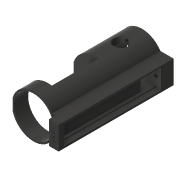
# Autodesk Inventor part: Holder for Fan
Saved by Autodesk Inventor 2017 (Build 210142000, 142)
## iProperties
Created: 2016-08-05
Part Number: Holder for Fan
Material: Generic
Document SubType Name: Modeling
Designer: ge937963
Density: 1 g/cm^3
Appearance: Smooth - Black
Mass: 19.5936 g
Surface Area: 136.055 cm^2
Volume: 19.5936 cm^3
Author: ge937963
Autodesk Inventor part; units mm, degrees
ref_plane "YZ Plane" through (0, 0, 0) normal (1, 0, 0) x (0, 1, 0)
ref_plane "XZ Plane" through (0, 0, 0) normal (0, 1, 0) x (-1, 0, 0)
sketch "Sketch1" plane through (0, 0, 0) normal (0, 0, 1) x (1, 0, 0)
  circle A0 centre (0, 0) radius 12.7
  circle A1 centre (0, 0) radius 9.525
  dimension "d0" = 25.4
  dimension "d1" = 19.05
  constraints: 2 centre point, 2 coincident
  measures "d0" diameter of A0
  measures "d1" diameter of A1
extrude "Extrusion1" add sketch "Sketch1" along normal blind 25.4 and the other way blind 12.7
sketch "Sketch2" plane through (0, 0, -12.7) normal (0, 0, -1) x (-1, 0, 0)
  circle A0 centre (0, 0) radius 12.7
  dimension "d6" = 25.4
  constraints: 1 centre point, 1 coincident
  measures "d6" diameter of A0
extrude "Extrusion2" add sketch "Sketch2" against normal blind 3.175
sketch "Sketch3" plane through (0, 0, -12.7) normal (0, 0, -1) x (-1, 0, 0)
  circle A0 centre (0, 0) radius 14.2875
  circle A1 centre (0, 0) radius 12.7
  dimension "d9" = 28.575
  constraints: 2 centre point, 2 coincident
  measures "d9" diameter of A0
extrude "Extrusion3" add sketch "Sketch3" against normal blind 66.675
sketch "Sketch4" plane through (0, 0, 0) normal (1, 0, 0) x (0, 1, 0)
  line L0 (-19.206, 6.35) -> (20.1125, 6.35)
  line L1 (20.1125, 6.35) -> (20.1125, 25.4)
  line L2 (20.1125, 25.4) -> (-19.206, 25.4)
  line L3 (-19.206, 25.4) -> (-19.206, 6.35)
  line L4 (14.2875, -12.7) -> (-14.2875, -12.7) projected
  point P0 (0, 0)
  dimension "d12" = 19.05
  dimension "d13" = 19.05
  constraints: 8 end point, 2 parallel, 1 horizontal, 1 perpendicular
  measures "d12" distance of L0.end L1.end
  measures "d13" distance from line of L4 L0.end
extrude "Extrusion4" cut sketch "Sketch4" along normal blind 2.54 and the other way blind 66.675
sketch "Sketch5" plane through (0, 0, 0) normal (1, 0, 0) x (0, 1, 0)
  line L0 (-1.5875, -17.2077) -> (1.5875, -17.2077) projected
  line L1 (-1.5875, -18.0015) -> (-1.5875, -16.414) projected
  line L2 (1.5875, -16.414) -> (-1.5875, -16.414) projected
  line L3 (1.5875, -16.414) -> (1.5875, -18.0015) projected
  line L4 (-1.5875, -18.0015) -> (1.5875, -18.0015) projected
  line L5 (-1.7071, -16.2944) -> (-1.7071, -18.121)
  line L6 (-1.7071, -18.121) -> (1.7071, -18.121)
  line L7 (1.7071, -18.121) -> (1.7071, -16.2944)
  line L8 (1.7071, -16.2944) -> (-1.7071, -16.2944)
  point P0 (0, 0)
  constraints: 8 end point, 3 other
extrude "Extrusion5" cut sketch "Sketch5" along normal blind 66.675 contours L1 L2 L3 L0 | L0 L3 L4 L1 | L8 L7 L6 L5
sketch "Sketch6" plane through (0, 0, 53.975) normal (0, 0, 1) x (1, 0, 0)
  line L0 (19.2175, 5.4663) -> (15.9155, 5.4663) projected
  line L1 (15.9155, 5.4663) -> (15.9155, -5.4557) projected
  line L2 (15.9155, -5.4557) -> (19.2175, -5.4557) projected
  line L3 (19.2175, -5.4557) -> (19.2175, 5.4663) projected
  line L4 (20.7415, -7.6147) -> (14.3915, -7.6147) projected
  line L5 (14.3915, -7.6147) -> (14.3915, 7.6253) projected
  line L6 (14.3915, 7.6253) -> (20.7415, 7.6253) projected
  line L7 (20.7415, 7.6253) -> (20.7415, -7.6147) projected
  point P0 (0, 0)
extrude "Extrusion6" add sketch "Sketch6" against normal blind 9.525
sketch "Sketch7" plane through (14.3915, -7.6147, 53.975) normal (-1, 0, 0) x (0, 0, 1)
  line L0 (0, 0) -> (0, 15.24) projected
  line L1 (0, 15.24) -> (-9.525, 15.24) projected
  line L2 (-9.525, 0) -> (-9.525, 15.24) projected
  line L3 (0, 0) -> (-9.525, 0) projected
  point P0 (-53.975, 7.6147)
extrude "Extrusion7" add sketch "Sketch7" along normal blind 2.54
sketch "Sketch8" plane through (0, 0, 53.975) normal (0, 0, 1) x (1, 0, 0)
  arc A0 (11.8515, 4.5641) -> (11.8515, -4.5641) centre (0, 0) ccw projected
  arc A1 (2.54, -12.4434) -> (2.54, 12.4434) centre (0, 0) ccw projected
  point P0 (0, -12.7)
  point P1 (0, 12.7)
extrude "Extrusion8" cut sketch "Sketch8" against normal blind 12.7
sketch "Sketch9" plane through (0, 0, 44.45) normal (0, 0, -1) x (-1, 0, 0)
  line L0 (-15.9155, 5.4663) -> (-15.9155, -5.4557) projected
  line L1 (-15.9155, -5.4557) -> (-19.2175, -5.4557) projected
  line L2 (-19.2175, -5.4557) -> (-19.2175, 5.4663) projected
  line L3 (-19.2175, 5.4663) -> (-15.9155, 5.4663) projected
  line L4 (-20.7415, -7.6147) -> (-12.0892, -7.6147) projected
  arc A0 (-12.0826, 7.6253) -> (-12.0892, -7.6147) centre (0, 0) ccw projected
  line L5 (-20.7415, 7.6253) -> (-12.0826, 7.6253) projected
  line L6 (-20.7415, 7.6253) -> (-20.7415, -7.6147) projected
extrude "Extrusion9" add sketch "Sketch9" along normal up to surface (57.15 mm away)
sketch "Sketch10" plane through (0, 0, -12.7) normal (0, 0, -1) x (-1, 0, 0)
  line L0 (-15.9155, 5.4663) -> (-15.9155, -5.4557) projected
  line L1 (-19.2175, -5.4557) -> (-19.2175, 5.4663) projected
  line L2 (-15.9155, 5.4663) -> (-19.2175, 5.4663)
  line L3 (-19.2175, 5.4663) -> (-19.2175, -5.4557)
  line L4 (-19.2175, -5.4557) -> (-15.9155, -5.4557)
  line L5 (-15.9155, -5.4557) -> (-15.9155, 5.4663)
  point P0 (0, 0)
  constraints: 8 end point, 2 parallel, 1 horizontal, 1 perpendicular
extrude "Extrusion10" add sketch "Sketch10" against normal blind 3.175
sketch "Sketch11" plane through (20.7415, -7.6147, 53.975) normal (1, 0, 0) x (0, 0, -1)
  line L0 (0, 15.24) -> (0, 0) projected
  line L1 (0, 0) -> (66.675, 0) projected
  line L2 (66.675, 15.24) -> (66.675, 0) projected
  line L3 (0, 15.24) -> (66.675, 15.24) projected
  line L4 (0, 1.27) -> (63.5, 1.27)
  line L5 (63.5, 1.27) -> (63.5, 13.97)
  line L6 (63.5, 13.97) -> (0, 13.97)
  line L7 (0, 13.97) -> (0, 1.27)
  point P0 (53.975, 7.6147)
  dimension "d28" = 0
  dimension "d29" = 1.27
  dimension "d30" = 1.27
  dimension "d31" = 63.5
  constraints: 8 end point, 2 parallel, 1 horizontal, 1 perpendicular
  measures "d28" distance between parallel lines of L0 L7
  measures "d29" distance between parallel lines of L1 L4
  measures "d30" distance between parallel lines of L3 L6
  measures "d31" distance of L5.end L6.end
extrude "Extrusion11" cut sketch "Sketch11" against normal blind 3.175 contours L6 L5 L4 L0
sketch "Sketch12" plane through (0, 0, 53.975) normal (0, 0, 1) x (1, 0, 0)
  line L0 (19.2175, 5.4663) -> (15.9155, 5.4663) projected
  line L1 (15.9155, 5.4663) -> (15.9155, -5.4557) projected
  line L2 (15.9155, -5.4557) -> (19.2175, -5.4557) projected
  line L3 (19.2175, -5.4557) -> (19.2175, 5.4663) projected
  line L4 (20.7415, -7.6147) -> (14.3915, -7.6147) projected
  line L5 (14.3915, -7.6147) -> (14.3915, 7.6253) projected
  line L6 (14.3915, 7.6253) -> (20.7415, 7.6253) projected
  line L7 (20.7415, 7.6253) -> (20.7415, -7.6147) projected
  line L8 (14.3915, -7.6147) -> (20.7415, -7.6147) projected
  line L9 (20.7415, -7.6147) -> (20.7415, 7.6253) projected
  line L10 (20.7415, 7.6253) -> (14.3915, 7.6253) projected
  line L11 (14.3915, 7.6253) -> (14.3915, -7.6147) projected
  circle A0 centre (17.5665, 3.8153) radius 0.762 projected
  circle A1 centre (17.5665, 1.2753) radius 0.762 projected
  circle A2 centre (17.5665, -1.2647) radius 0.762 projected
  circle A3 centre (17.5665, -3.8047) radius 0.762 projected
  line L12 (17.5665, -6.3447) -> (17.5665, -5.4557) projected
  line L13 (17.5665, -5.4557) -> (17.5665, -6.3447) projected
  line L14 (17.5665, 6.3553) -> (17.5665, 5.4663) projected
  line L15 (17.5665, 5.4663) -> (17.5665, 6.3553) projected
  line L16 (17.5665, -5.4557) -> (15.9155, -5.4557) projected
  line L17 (17.5665, -5.4557) -> (15.9155, -5.4557)
  line L18 (15.9155, -5.4557) -> (15.9155, 5.4663) projected
  line L19 (15.9155, -5.4557) -> (15.9155, 5.4663)
  line L20 (15.9155, 5.4663) -> (17.5665, 5.4663)
  line L21 (17.5665, 6.3553) -> (17.5665, 5.4663) projected
  line L22 (17.5665, 6.3553) -> (20.7415, 6.3553)
  line L23 (20.7415, -6.3447) -> (17.5665, -6.3447)
  line L24 (20.7415, 7.6253) -> (20.7415, -7.6147) projected
  line L25 (17.5665, -5.4557) -> (17.5665, -6.3447) projected
  line L26 (17.5665, -5.4557) -> (15.9155, -5.4557)
  line L27 (20.7415, -6.3447) -> (20.7415, -7.6147)
  point P0 (0, 0)
  constraints: 14 end point, 5 perpendicular, 1 collinear, 1 parallel
extrude "Extrusion12" add sketch "Sketch12" along normal up to surface (4.1732 mm away) contours L0 L1 L2 L12 L23 L7 L4 L5 L6 L22 L14
sketch "Sketch13" plane through (15.9155, -5.4557, -9.525) normal (1, 0, 0) x (0, 0, -1)
  line L0 (3.175, -2.159) -> (-67.6732, -2.159) projected
  line L1 (-66.6572, -2.159) -> (-67.6732, -2.159)
  line L2 (-67.6732, -2.159) -> (-67.6732, 13.081)
  line L3 (-67.6732, 13.081) -> (-66.6572, 13.081)
  line L4 (-66.6572, 13.081) -> (-66.6572, -2.159)
  line L5 (-66.6572, 9.7155) -> (-72.4992, 9.7155)
  point P0 (-9.525, 5.4557)
  point P1 (-67.1652, -2.159)
  point P2 (-67.1652, 13.081)
  point P3 (-67.6732, 5.461)
  constraints: 10 end point, 3 midpoint, 2 horizontal, 2 horizontal alignment, 2 parallel, 2 vertical alignment, 1 perpendicular, 1 point on line, 2 other
extrude "Extrusion13" add sketch "Sketch13" along normal up to surface (4.826 mm away)
sketch "Sketch14" plane through (14.3915, 7.6253, 58.1482) normal (0, 0, 1) x (1, 0, 0)
  circle A0 centre (3.175, -3.81) radius 0.762 projected
  circle A1 centre (3.175, -6.35) radius 0.762 projected
  circle A2 centre (3.175, -8.89) radius 0.762 projected
  circle A3 centre (3.175, -11.43) radius 0.762 projected
  point P0 (-14.3915, -7.6253)
extrude "Extrusion14" cut sketch "Sketch14" against normal blind 3.175
sketch "Sketch15" plane through (17.5665, -7.6147, 53.975) normal (1, 0, 0) x (0, 0, -1)
  line L0 (2.1768, 15.24) -> (5.7328, 15.24) projected
  line L1 (2.1768, 0) -> (2.1768, 15.24) projected
  line L2 (5.7328, 0) -> (2.1768, 0) projected
  line L3 (5.7328, 15.24) -> (5.7328, 0) projected
  line L4 (-3.1572, 13.081) -> (5.7328, 13.081) projected
  line L5 (-3.1572, 2.159) -> (5.7328, 2.159) projected
  line L6 (63.5, 1.27) -> (-3.1572, 1.27) projected
  line L7 (-3.1572, 2.159) -> (5.7328, 2.159)
  line L8 (5.7328, 2.159) -> (5.7328, 1.27)
  line L9 (5.7328, 1.27) -> (-3.1572, 1.27)
  line L10 (-3.1572, 1.27) -> (-3.1572, 2.159)
  line L11 (-3.1572, 13.081) -> (-3.1572, 2.159) projected
  line L12 (-3.1572, 13.97) -> (63.5, 13.97) projected
  line L13 (-3.1572, 13.081) -> (5.7328, 13.081)
  line L14 (5.7328, 13.081) -> (5.7328, 13.97)
  line L15 (5.7328, 13.97) -> (-3.1572, 13.97)
  line L16 (-3.1572, 13.97) -> (-3.1572, 13.081)
  point P0 (53.975, 7.6147)
  constraints: 16 end point, 4 parallel, 4 point on line, 2 perpendicular, 1 horizontal
extrude "Extrusion15" add sketch "Sketch15" along normal up to surface (3.175 mm away) contours L12 L3 L4 L1 | L1 L4 L16 L12 | L5 L3 L6 L1 | L1 L6 L10 L5
sketch "Sketch16" plane through (15.9155, -5.4557, 57.1322) normal (0, 0, -1) x (-1, 0, 0)
  line L0 (-4.826, 10.922) -> (-4.826, 0) projected
  line L1 (-4.826, 10.922) -> (0, 10.922) projected
  line L2 (-4.826, 0) -> (-3.302, 0)
  line L3 (-3.302, 0) -> (-3.302, 10.922)
  line L4 (-3.302, 10.922) -> (-4.826, 10.922)
  line L5 (-4.826, 10.922) -> (-4.826, 0)
  line L6 (-3.302, 10.922) -> (-3.302, 0) projected
  point P0 (15.9155, 5.4557)
  point P1 (-3.302, 5.461)
  point P2 (-4.826, 11.811)
  point P3 (-4.826, -0.889)
  point P4 (-1.651, 10.922)
  constraints: 8 end point, 2 parallel, 1 collinear, 1 horizontal, 1 midpoint, 1 perpendicular, 1 point on line, 1 vertical alignment
ref_plane "Work Plane1" through (14.3915, -7.6147, 54.5922) normal (0, 0, -1) x (0, 1, 0)
extrude "Extrusion16" add sketch "Sketch16" along normal up to surface (2.54 mm away)
sketch "Sketch17" plane through (15.9155, -5.4557, -9.525) normal (1, 0, 0) x (0, 0, -1)
  line L0 (0, 2.2807) -> (-3.175, 2.2807)
  line L1 (-3.175, 2.2807) -> (-3.175, 8.6307)
  line L2 (-3.175, 8.6307) -> (0, 8.6307)
  line L3 (0, 8.6307) -> (0, 2.2807)
  line L4 (-66.6572, 10.922) -> (-66.6572, 0) projected
  line L5 (-66.6572, 0) -> (0, 0) projected
  line L6 (0, 0) -> (0, 10.922) projected
  line L7 (0, 10.922) -> (-66.6572, 10.922) projected
  point P0 (-9.525, 5.4557)
  point P1 (-3.175, 5.4557)
  dimension "d44" = 6.35
  dimension "d45" = 3.175
  dimension "d46" = 0
  constraints: 8 end point, 2 parallel, 1 horizontal, 1 horizontal alignment, 1 midpoint, 1 perpendicular
  measures "d44" distance of L0.end L1.end
  measures "d45" distance of L0.start L0.end
  measures "d46" distance between parallel lines of L6 L3
extrude "Extrusion17" cut sketch "Sketch17" against normal blind 12.7 contours L0 L1 L2 L3
sketch "Sketch18" plane through (0, 0, -12.7) normal (0, 0, -1) x (-1, 0, 0)
  line L0 (16.7262, -5.3355) -> (13.6621, -5.3355)
  line L1 (13.6621, -5.3355) -> (13.6621, 5.7627)
  line L2 (13.6621, 5.7627) -> (16.7262, 5.7627)
  line L3 (16.7262, 5.7627) -> (16.7262, -5.3355)
  point P0 (0, 0)
  constraints: 8 end point, 2 parallel, 1 horizontal, 1 perpendicular
extrude "Extrusion18" cut sketch "Sketch18" against normal through all
sketch "Sketch19" plane through (0, 0, 53.975) normal (0, 0, 1) x (1, 0, 0)
  circle A0 centre (0, 0) radius 13.208
  dimension "d51" = 26.416
  constraints: 1 centre point, 1 coincident
  measures "d51" diameter of A0
extrude "Extrusion19" cut sketch "Sketch19" against normal up to surface (28.575 mm away)
sketch "Sketch20" plane through (0, 0, 25.4) normal (0, 0, 1) x (1, 0, 0)
  circle A0 centre (0, 0) radius 10.033
  dimension "d54" = 20.066
  constraints: 1 centre point, 1 coincident
  measures "d54" diameter of A0
extrude "Extrusion20" cut sketch "Sketch20" against normal up to surface (34.925 mm away)
chamfer "Chamfer1" distance 3.175 angle 45 2 edges at (7.9418, 6.131, 25.4) (7.9418, -6.131, 25.4)
sketch "Sketch21" plane through (0, 0, -12.7) normal (0, 0, -1) x (-1, 0, 0)
  line L0 (13.6621, -4.1808) -> (13.6621, 4.1808) projected
  arc A0 (13.6621, 4.1808) -> (-12.0826, 7.6253) centre (0, 0) ccw projected
  line L1 (-12.0826, 7.6253) -> (-20.7415, 7.6253) projected
  line L2 (-20.7415, 7.6253) -> (-20.7415, -7.6147) projected
  line L3 (-20.7415, -7.6147) -> (-12.0892, -7.6147) projected
  arc A1 (-12.0892, -7.6147) -> (13.6621, -4.1808) centre (0, 0) ccw projected
extrude "Extrusion21" add sketch "Sketch21" along normal blind 5.08
chamfer "Chamfer2" distance 3.175 angle 45 2 edges at (9.9033, 1.6083, -6.35) (9.9033, -1.6083, -6.35)
sketch "Sketch22" plane through (0, 0, 53.975) normal (0, 0, 1) x (1, 0, 0)
  line L0 (-34.0528, 26.6129) -> (2.54, 26.6129)
  line L1 (2.54, 26.6129) -> (2.54, -32.6193)
  line L2 (2.54, -32.6193) -> (-34.0528, -32.6193)
  line L3 (-34.0528, -32.6193) -> (-34.0528, 26.6129)
  line L4 (2.54, -9.7062) -> (2.54, -12.9615) projected
  arc A0 (2.54, -12.9615) -> (2.54, 12.9615) centre (0, 0) ccw projected
  line L5 (2.54, 12.9615) -> (2.54, 9.7062) projected
  arc A1 (2.54, -9.7062) -> (2.54, 9.7062) centre (0, 0) ccw projected
  constraints: 8 end point, 2 parallel, 1 horizontal, 1 perpendicular, 1 vertical alignment
extrude "Extrusion22" [suppressed]
sketch "Sketch23" plane through (2.54, 0, 0) normal (-1, 0, 0) x (0, 0, 1)
  line L0 (13.6509, -14.0599) -> (12.0634, -14.0599)
  line L1 (12.0634, -14.0599) -> (12.0634, -14.0599)
  line L2 (12.0634, -14.0599) -> (13.6509, -14.0599)
  line L3 (13.6509, -14.0599) -> (13.6509, -14.0599)
  line L4 (13.6509, 3.556) -> (13.6509, -3.556) projected
  point P0 (0, 0)
  point P1 (6.35, 14.0599)
  point P2 (53.975, 14.0599)
  point P3 (6.35, -14.0599)
  dimension "d69" = 1.5875
  constraints: 8 end point, 2 equal length, 1 horizontal, 1 horizontal alignment, 1 perpendicular, 1 vertical alignment, 2 other
  measures "d69" distance between parallel lines of L1 L3
extrude "Extrusion23" [suppressed]
sketch "Sketch24" plane through (0, 0, -17.78) normal (0, 0, -1) x (-1, 0, 0)
  arc A0 (-2.54, 14.0599) -> (-12.0826, 7.6253) centre (0, 0) ccw projected
  line L0 (-21.59, 14.0599) -> (-2.54, 14.0599) projected
  line L1 (-21.59, -14.0599) -> (-21.59, 14.0599) projected
  line L2 (-21.59, -14.0599) -> (-2.54, -14.0599) projected
  arc A1 (-12.0892, -7.6147) -> (-2.54, -14.0599) centre (0, 0) ccw projected
  line L3 (-20.7415, -7.6147) -> (-12.0892, -7.6147) projected
  line L4 (-20.7415, -6.3447) -> (-20.7415, -7.6147) projected
  line L5 (-17.5665, -6.3447) -> (-20.7415, -6.3447) projected
  line L6 (-17.5665, -5.4557) -> (-17.5665, -6.3447) projected
  line L7 (-15.9155, -5.4557) -> (-17.5665, -5.4557) projected
  line L8 (-15.9155, 5.4663) -> (-15.9155, -5.4557) projected
  line L9 (-17.5665, 5.4663) -> (-15.9155, 5.4663) projected
  line L10 (-17.5665, 6.3553) -> (-17.5665, 5.4663) projected
  line L11 (-20.7415, 6.3553) -> (-17.5665, 6.3553) projected
  line L12 (-20.7415, 7.6253) -> (-20.7415, 6.3553) projected
  line L13 (-12.0826, 7.6253) -> (-20.7415, 7.6253) projected
  line L14 (-2.54, 9.7062) -> (-2.54, 14.0599) projected
  arc A2 (-2.54, 9.7062) -> (-2.54, -9.7062) centre (0, 0) ccw projected
  line L15 (-2.54, -14.0599) -> (-2.54, -9.7062) projected
  line L16 (-2.54, -14.0599) -> (16.51, -14.0599) projected
  line L17 (16.51, 14.0599) -> (16.51, -14.0599) projected
  line L18 (-2.54, 14.0599) -> (16.51, 14.0599) projected
  arc A3 (-12.0892, -7.6147) -> (13.6621, -4.1808) centre (0, 0) ccw projected
  line L19 (13.6621, -4.1808) -> (13.6621, 4.1808) projected
  arc A4 (13.6621, 4.1808) -> (-12.0826, 7.6253) centre (0, 0) ccw projected
  arc A5 (13.6621, 4.1808) -> (-2.54, 14.0599) centre (0, 0) ccw projected
  arc A6 (-2.54, -14.0599) -> (13.6621, -4.1808) centre (0, 0) ccw projected
  arc A7 (-2.54, -14.0599) -> (13.6621, -4.1808) centre (0, 0) ccw projected
  arc A8 (-12.0892, -7.6147) -> (13.6621, -4.1808) centre (0, 0) ccw projected
  arc A9 (-12.0892, -7.6147) -> (13.6621, -4.1808) centre (0, 0) ccw projected
  arc A10 (13.6621, 4.1808) -> (-12.0826, 7.6253) centre (0, 0) ccw projected
  arc A11 (13.6621, 4.1808) -> (-2.54, 14.0599) centre (0, 0) ccw projected
extrude "Extrusion24" [suppressed]
sketch "Sketch25" plane through (2.54, 9.7062, 12.0634) normal (0, 0, -1) x (-1, 0, 0)
  line L0 (16.2021, -13.8869) -> (16.2021, -5.5254) projected
  arc A0 (-9.5492, -17.3209) -> (16.2021, -13.8869) centre (2.54, -9.7062) ccw projected
  arc A1 (16.2021, -5.5254) -> (-9.5426, -2.0809) centre (2.54, -9.7062) ccw projected
  arc A2 (16.2021, -5.5254) -> (0, 4.3538) centre (2.54, -9.7062) ccw projected
  line L1 (2.2697, 4.5788) -> (24.3306, 17.5594)
  line L2 (24.3306, 17.5594) -> (25.4016, -34.733)
  line L3 (25.4016, -34.733) -> (2.2697, -23.9911)
  arc A3 (0, -23.7661) -> (16.2021, -13.8869) centre (2.54, -9.7062) ccw projected
  point P0 (2.54, -9.7062)
  constraints: 6 end point, 4 point on circle
extrude "Extrusion25" [suppressed]
sketch "Sketch26" plane through (2.54, -14.0599, 13.6509) normal (0, 0, 1) x (1, 0, 0)
  circle A0 centre (-2.54, 14.0599) radius 2.7 projected
  circle A1 centre (-2.54, 14.0599) radius 3.556 projected
  circle A2 centre (-2.54, 14.0599) radius 3.6
  point P0 (-2.54, 14.0599)
  dimension "d76" = 7.2
  constraints: 1 centre point, 1 coincident
  measures "d76" diameter of A2
extrude "Extrusion26" [suppressed]
sketch "Sketch27" plane through (0, 0, 53.975) normal (0, 0, 1) x (1, 0, 0)
  line L0 (-25.6623, -24.0934) -> (14.3915, -24.0934)
  line L1 (14.3915, -24.0934) -> (14.3915, 32.9463)
  line L2 (14.3915, 32.9463) -> (-25.6623, 32.9463)
  line L3 (-25.6623, 32.9463) -> (-25.6623, -24.0934)
  line L4 (14.3915, -7.6147) -> (14.3915, 7.6253) projected
  point P0 (0, 0)
  constraints: 8 end point, 2 parallel, 1 horizontal, 1 perpendicular, 1 vertical alignment
extrude "Extrusion27" [suppressed]
sketch "Sketch28" plane through (2.54, 0, 0) normal (-1, 0, 0) x (0, 0, 1)
  line L0 (13.6509, 31.1243) -> (12.0634, 31.1243)
  line L1 (12.0634, 31.1243) -> (12.0634, -32.0641)
  line L2 (12.0634, -32.0641) -> (13.6509, -32.0641)
  line L3 (13.6509, -32.0641) -> (13.6509, 31.1243)
  line L4 (13.6509, 3.556) -> (13.6509, -3.556) projected
  point P0 (0, 0)
  dimension "d81" = 1.5875
  constraints: 8 end point, 2 parallel, 1 horizontal, 1 perpendicular, 1 vertical alignment
  measures "d81" distance of L2.end L1.end
extrude "Extrusion28" add sketch "Sketch28" along normal mid plane 76.2
sketch "Sketch29" plane through (40.64, -32.0641, 12.0634) normal (0, 0, -1) x (-1, 0, 0)
  line L0 (19.8985, 39.6894) -> (19.8985, 24.4494) projected
  line L1 (19.8985, 24.4494) -> (28.5508, 24.4494) projected
  arc A0 (28.5508, 24.4494) -> (54.3021, 27.8834) centre (40.64, 32.0641) ccw projected
  line L2 (54.3021, 27.8834) -> (54.3021, 36.2449) projected
  arc A1 (54.3021, 36.2449) -> (28.5574, 39.6894) centre (40.64, 32.0641) ccw projected
  line L3 (28.5574, 39.6894) -> (19.8985, 39.6894) projected
  line L4 (117.3685, -15.5251) -> (-29.6456, -15.5251)
  line L5 (-29.6456, -15.5251) -> (-29.6456, 75.2605)
  line L6 (-29.6456, 75.2605) -> (117.3685, 75.2605)
  line L7 (117.3685, 75.2605) -> (117.3685, -15.5251)
  constraints: 8 end point, 2 parallel, 1 horizontal, 1 perpendicular
extrude "Extrusion29" cut sketch "Sketch29" against normal through all
sketch "Sketch30" plane through (2.54, -14.0599, 13.6509) normal (0, 0, 1) x (1, 0, 0)
  circle A0 centre (-2.54, 14.0599) radius 3.6
  dimension "d86" = 7.2
  constraints: 1 centre point, 1 coincident
  measures "d86" diameter of A0
extrude "Extrusion30" cut sketch "Sketch30" against normal blind 1.5875
sketch "Sketch31" plane through (-13.6621, -4.1808, 6.35) normal (0, 0, 1) x (1, 0, 0)
  arc A0 (16.2021, 13.8869) -> (16.2021, -5.5254) centre (13.6621, 4.1808) ccw projected
  line L0 (16.2021, 13.8869) -> (16.2021, 18.2407) projected
  arc A1 (16.2021, 18.2407) -> (0, 8.3615) centre (13.6621, 4.1808) ccw projected
  line L1 (0, 8.3615) -> (0, 0) projected
  arc A2 (0, 0) -> (16.2021, -9.8791) centre (13.6621, 4.1808) ccw projected
  line L2 (16.2021, -9.8791) -> (16.2021, -5.5254) projected
extrude "Extrusion31" add sketch "Sketch31" along normal up to surface (5.7134 mm away)
sketch "Sketch32" plane through (-13.6621, -4.1808, 53.975) normal (-1, 0, 0) x (0, 0, 1)
  line L0 (-35.8106, 34.7045) -> (-9.525, 34.7045)
  line L1 (-9.525, 34.7045) -> (-9.525, -32.5226)
  line L2 (-9.525, -32.5226) -> (-35.8106, -32.5226)
  line L3 (-35.8106, -32.5226) -> (-35.8106, 34.7045)
  line L4 (0, 8.3615) -> (0, 18.4683) projected
  point P0 (-53.975, 4.1808)
  point P1 (0, 11.806)
  dimension "d91" = 9.525
  constraints: 8 end point, 2 parallel, 1 horizontal, 1 perpendicular
  measures "d91" distance between parallel lines of L1 L4
extrude "Extrusion32" cut sketch "Sketch32" against normal up to surface (16.2021 mm away)
sketch "Sketch33" plane through (17.5665, 6.3553, 13.6509) normal (0, 0, 1) x (1, 0, 0)
  line L0 (3.175, -12.7) -> (3.175, 0) projected
  line L1 (0, 0) -> (3.175, 0) projected
  line L2 (0, -0.889) -> (0, 0) projected
  line L3 (-1.651, -0.889) -> (0, -0.889) projected
  line L4 (-1.651, -11.811) -> (-1.651, -0.889) projected
  line L5 (0, -11.811) -> (-1.651, -11.811) projected
  line L6 (0, -12.7) -> (0, -11.811) projected
  line L7 (3.175, -12.7) -> (0, -12.7) projected
  point P0 (-17.5665, -6.3553)
extrude "Extrusion33" cut sketch "Sketch33" against normal blind 1.5875
sketch "Sketch34" plane through (0, 0, -17.78) normal (0, 0, -1) x (-1, 0, 0)
  arc A0 (-9.5174, -3.175) -> (-9.5174, 3.175) centre (0, 0) ccw projected
  line L0 (-15.9155, -3.175) -> (-9.5174, -3.175) projected
  line L1 (-15.9155, -5.4557) -> (-15.9155, -3.175) projected
  line L2 (-17.5665, -5.4557) -> (-15.9155, -5.4557) projected
  line L3 (-17.5665, -5.4557) -> (-17.5665, -6.3447) projected
  line L4 (-20.7415, -6.3447) -> (-17.5665, -6.3447) projected
  line L5 (-20.7415, 6.3553) -> (-20.7415, -6.3447) projected
  line L6 (-20.7415, 6.3553) -> (-17.5665, 6.3553) projected
  line L7 (-17.5665, 6.3553) -> (-17.5665, 5.4663) projected
  line L8 (-15.9155, 5.4663) -> (-17.5665, 5.4663) projected
  line L9 (-15.9155, 3.175) -> (-15.9155, 5.4663) projected
  line L10 (-15.9155, 3.175) -> (-9.5174, 3.175) projected
  circle A1 centre (0, 0) radius 10.033
  constraints: 1 coincident, 3 other
extrude "Extrusion34" cut sketch "Sketch34" against normal blind 12.7 contours A1 A0
sketch "Sketch35" plane through (12.0892, -7.6147, 53.975) normal (0, -1, 0) x (1, 0, 0)
  line L0 (-18.2222, -43.8338) -> (-5.9562, -43.8338)
  line L1 (-5.9562, -43.8338) -> (-5.9562, -52.0554)
  line L2 (-5.9562, -52.0554) -> (-18.2222, -52.0554)
  line L3 (-18.2222, -52.0554) -> (-18.2222, -43.8338)
  line L4 (-15.6892, -40.3241) -> (-15.6892, -41.9116) projected
  line L5 (-8.4892, -40.3241) -> (-8.4892, -41.9116) projected
  line L6 (-12.0892, -43.8338) -> (-15.6892, -41.9116) construction
  line L7 (-12.0892, -43.8338) -> (-8.4892, -41.9116) construction
  point P0 (-12.0892, -53.975)
  constraints: 12 end point, 2 parallel, 1 equal length, 1 horizontal, 1 midpoint, 1 perpendicular
extrude "Extrusion35" [suppressed]
sketch "Sketch36" plane through (15.9155, -3.175, -6.35) normal (0, 0, -1) x (-1, 0, 0)
  line L0 (3.0948, 0) -> (6.3981, 0) projected
  arc A0 (6.3981, 6.35) -> (6.3981, 0) centre (15.9155, 3.175) ccw projected
  line L1 (6.3981, 6.35) -> (3.0948, 6.35) projected
  arc A1 (3.0948, 6.35) -> (3.0948, 0) centre (15.9155, 3.175) ccw projected
extrude "Extrusion36" cut sketch "Sketch36" along normal blind 12.7
sketch "Sketch37" plane through (0, 0, -17.78) normal (0, 0, -1) x (-1, 0, 0)
  circle A0 centre (0, -12.1603) radius 1.27
  circle A1 centre (0, 12.1583) radius 1.27
  circle A2 centre (-17.5665, 0.0053) radius 1.27
  circle A3 centre (0, 0) radius 10.033 projected
  line L0 (0, -10.033) -> (0, -14.2875) construction
  arc A4 (-12.0892, -7.6147) -> (13.6621, -4.1808) centre (0, 0) ccw projected
  line L1 (0, 10.029) -> (0, 14.2875) construction
  arc A5 (13.6621, 4.1808) -> (-12.0826, 7.6253) centre (0, 0) ccw projected
  line L2 (-20.7415, 7.6253) -> (-20.7415, -7.6147) projected
  point P0 (0, -12.1603)
  point P1 (0, 12.1583)
  dimension "d102" = 2.54
  dimension "d103" = 2.54
  dimension "d104" = 2.54
  dimension "d105" = 3.175
  constraints: 4 end point, 3 centre point, 2 coincident, 2 midpoint, 2 point on circle, 2 point on line, 1 vertical, 1 vertical alignment, 1 other
  measures "d102" diameter of A0
  measures "d103" diameter of A1
  measures "d104" diameter of A2
  measures "d105" distance from line of A2.centre L2
extrude "Extrusion37" cut sketch "Sketch37" against normal blind 12.7 contours A0 | A1 | A2
sketch "Sketch38" plane through (15.9155, -5.4557, 57.1322) normal (1, 0, 0) x (0, 0, -1)
  line L0 (66.6572, 8.6307) -> (66.6572, 10.922) projected
  line L1 (8.89, 0) -> (66.6572, 0) projected
  line L2 (66.6572, 10.922) -> (58.114, 10.922)
  line L3 (58.114, 10.922) -> (58.114, 0)
  line L4 (58.114, 0) -> (66.6572, 0)
  line L5 (66.6572, 0) -> (66.6572, 10.922)
  point P0 (57.1322, 5.4557)
  constraints: 8 end point, 2 parallel, 1 horizontal, 1 perpendicular, 1 point on line
extrude "Extrusion38" cut sketch "Sketch38" against normal blind 12.7
sketch "Sketch39" plane through (0, 0, 0) normal (0, 1, 0) x (-1, 0, 0)
  circle A0 centre (0, -3.2548) radius 3.429 projected
  circle A1 centre (0, -3.2548) radius 4.6672
  point P0 (0, 0)
  constraints: 1 centre point, 1 coincident
extrude "Extrusion39" cut sketch "Sketch39" against normal blind 25.4 contours A0 | A1
sketch "Sketch40" plane through (0, 0, 0) normal (0, 1, 0) x (-1, 0, 0)
  spline S0 degree 8 poles (4.6672, -3.2548) (4.6672, -2.7831) (4.6127, -2.3128) (4.5044, -1.8475) (4.3413, -1.3908) (4.122, -0.9471) (3.8439, -0.5224) (3.5039, -0.1246) (2.8151, 0.4872) (2.4917, 0.7271) (2.1308, 0.9438) (1.7357, 1.1285) (1.3108, 1.2735) (0.8622, 1.3723) (0.3964, 1.4198) (-0.6626, 1.4019) (-1.2216, 1.309) (-1.7455, 1.1448) (-2.2265, 0.9208) (-2.659, 0.6485) (-3.0395, 0.3399) (-3.3667, 0.0074) (-3.9036, -0.6625) (-4.1248, -1.0071) (-4.3071, -1.3652) (-4.4517, -1.7334) (-4.5595, -2.1087) (-4.6313, -2.4888) (-4.6672, -2.8716) (-4.6672, -3.7266) (-4.6127, -4.1969) (-4.5044, -4.6622) (-4.3413, -5.1189) (-4.122, -5.5625) (-3.8439, -5.9873) (-3.5039, -6.385) (-2.8151, -6.9969) (-2.4917, -7.2368) (-2.1308, -7.4535) (-1.7357, -7.6382) (-1.3108, -7.7831) (-0.8622, -7.882) (-0.3964, -7.9294) (0.5838, -7.9129) (1.0728, -7.8421) (1.5378, -7.7158) (1.9726, -7.5411) (2.372, -7.3258) (2.7321, -7.0785) (3.051, -6.8088) (3.6719, -6.1773) (3.9617, -5.7985) (4.1995, -5.3989) (4.3875, -4.9844) (4.5274, -4.5594) (4.6205, -4.1275) (4.6672, -3.6917) (4.6672, -3.2548) knots 0 0 0 0 0 0 0 0 0 0.147026 0.147026 0.147026 0.147026 0.147026 0.147026 0.147026 0.250409 0.250409 0.250409 0.250409 0.250409 0.250409 0.250409 0.377395 0.377395 0.377395 0.377395 0.377395 0.377395 0.377395 0.498096 0.498096 0.498096 0.498096 0.498096 0.498096 0.498096 0.646671 0.646671 0.646671 0.646671 0.646671 0.646671 0.646671 0.751144 0.751144 0.751144 0.751144 0.751144 0.751144 0.751144 0.862163 0.862163 0.862163 0.862163 0.862163 0.862163 0.862163 1 1 1 1 1 1 1 1 1 projected
  point P0 (0, 0)
  constraints: 1 other
extrude "Extrusion40" cut sketch "Sketch40" along normal blind 25.4
sketch "Sketch41" plane through (17.5665, -6.3447, 48.2422) normal (0, 0, -1) x (-1, 0, 0)
  line L0 (-3.175, 0.889) -> (-3.175, 0) projected
  line L1 (0, 0) -> (-3.175, 0) projected
  line L2 (0, 0.889) -> (0, 0) projected
  line L3 (0, 0.889) -> (-3.175, 0.889) projected
  line L4 (-3.175, 12.7) -> (-3.175, 11.811) projected
  line L5 (0, 11.811) -> (-3.175, 11.811) projected
  line L6 (0, 12.7) -> (0, 11.811) projected
  line L7 (-3.175, 12.7) -> (0, 12.7) projected
  point P0 (17.5665, 6.3447)
extrude "Extrusion41" cut sketch "Sketch41" against normal up to surface (6.35 mm away)
body "Solid1"
